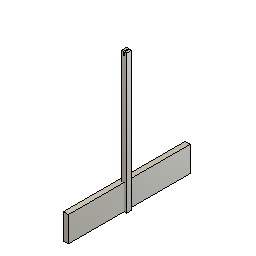
Oregon+Badminton (Autodesk Fusion 360 design; units mm, degrees)
Autodesk Fusion 360 part; units mm, degrees
sketch "Sketch1" plane through (0, 0, 0) normal (0, 0, 1) x (1, 0, 0)
  line L0 (0, 0) -> (914.4, 0)
  line L1 (914.4, 0) -> (914.4, 190.5)
  line L2 (914.4, 190.5) -> (0, 190.5)
  line L3 (0, 190.5) -> (0, 0)
  dimension "d1" = 914.4
  dimension "d2" = 190.5
  constraint horizontal L0
  constraint vertical L1
  constraint horizontal L2
  constraint vertical L3
  constraint coincident L0.start L3.end
  measures "d1" distance of L0.start L0.end
  measures "d2" distance of L0.start L2.end
extrude "Extrude1" add sketch "Sketch1" along normal blind 38.1 makes body 1
copy_body "Body->Comp1" bodies 1 removing the originals makes body 2 in component "Base"
sketch "Sketch2" plane through (0, 0, 0) normal (0, 0, 1) x (1, 0, 0)
  line L0 (-396.24, 523.24) -> (-358.14, 523.24)
  line L1 (-358.14, 523.24) -> (-358.14, -518.16)
  line L2 (-358.14, -518.16) -> (-396.24, -518.16)
  line L3 (-396.24, -518.16) -> (-396.24, 523.24)
  dimension "d5" = 38.1
  dimension "d6" = 1041.4
  constraint horizontal L0
  constraint vertical L1
  constraint horizontal L2
  constraint vertical L3
  measures "d5" distance of L0.start L0.end
  measures "d6" distance of L0.start L2.end
extrude "Extrude2" add sketch "Sketch2" along normal blind 38.1 separate body makes body 3
copy_body "Body->Comp2" bodies 3 removing the originals makes body 4 in component "Suport"
sketch "Sketch3" plane through (0, 523.24, 0) normal (0, 1, 0) x (-1, 0, 0)
  line L0 (358.14, 0) -> (396.24, 0)
  line L1 (396.24, 0) -> (396.24, 38.1)
  line L2 (396.24, 38.1) -> (358.14, 38.1)
  line L3 (358.14, 38.1) -> (358.14, 0)
  line L4 (374.015, 38.1) -> (380.365, 38.1)
  line L5 (380.365, 38.1) -> (380.365, 0)
  line L6 (380.365, 0) -> (374.015, 0)
  line L7 (374.015, 0) -> (374.015, 38.1)
  dimension "d13" = 6.35
  constraint horizontal L4
  constraint vertical L5
  constraint horizontal L6
  constraint vertical L7
  constraint coincident L2 L4.start
  constraint midpoint L2 L4
  measures "d13" distance of L4.start L4.end
extrude "Extrude1'" cut sketch "Sketch3" against normal blind 25.4 contours L0 L2 L4 L5 L6 L7 bodies 4 in component "Suport"
component "Base" placed x (0, 0, -1) y (0, 1, 0) z (1, 0, 0) at (-415.29, -518.16, 457.2)
component "Suport" placed x (1, 0, 0) y (0, 1, 0) z (0, 0, 1) at (0, 0, 0)
